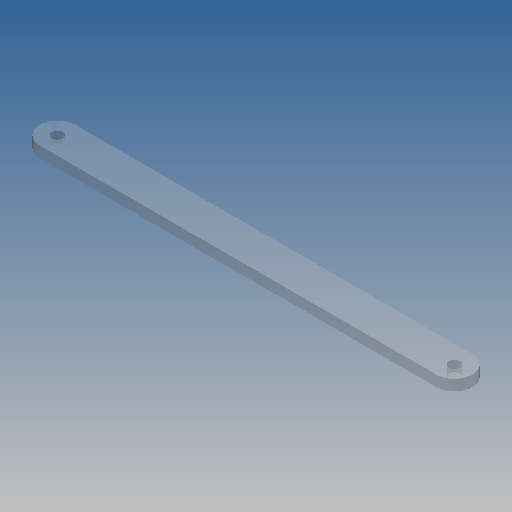
# Autodesk Inventor part: Handle
Saved by Autodesk Inventor 2017 (Build 210142000, 142)
## iProperties
Created: 2016-11-22
Part Number: Handle
Material: Polycarbonate, Clear
Document SubType Name: Modeling
Designer: James Yelland
Density: 1.2 g/cm^3
Appearance: Polycarbonate - Clear
Author: James Yelland
Autodesk Inventor part; units mm, degrees
ref_plane "YZ Plane" through (0, 0, 0) normal (1, 0, 0) x (0, 1, 0)
ref_plane "XZ Plane" through (0, 0, 0) normal (0, 1, 0) x (-1, 0, 0)
ref_plane "XY Plane" through (0, 0, 0) normal (0, 0, 1) x (1, 0, 0)
sketch "Sketch1" plane through (0, 0, 0) normal (0, 1, 0) x (-1, 0, 0)
  circle A0 centre (-55.4009, 75.9203) radius 1.6
  circle A1 centre (55.3868, 75.9203) radius 1.6
  arc A2 (55.3868, 70.9203) -> (55.3868, 80.9203) centre (55.3868, 75.9203) ccw
  line L0 (55.3868, 75.9203) -> (55.3868, 70.9203) construction
  line L1 (55.3868, 75.9203) -> (60.3868, 75.9203) construction
  line L2 (55.3868, 75.9203) -> (55.3868, 80.9203) construction
  arc A3 (-55.4009, 80.9203) -> (-55.4009, 70.9203) centre (-55.4009, 75.9203) ccw
  line L3 (-55.4009, 75.9203) -> (-50.4009, 75.9203) construction
  line L4 (-55.4009, 75.9203) -> (-55.4009, 80.9203) construction
  line L5 (-55.4009, 80.9203) -> (55.3868, 80.9203)
  line L6 (55.3868, 70.9203) -> (-55.4009, 70.9203)
  dimension "d13" = 5
  dimension "d14" = 90
  dimension "d15" = 180
  dimension "d16" = 5
  constraints: 14 end point, 4 centre point, 4 point on circle, 3 horizontal, 2 coincident, 1 perpendicular
  measures "d13" radius of A2
  measures "d14" angle of L0 L1
  measures "d15" angle of L0 L2
  measures "d16" radius of A3
extrude "Extrusion1" add sketch "Sketch1" along normal blind 3
body "Solid1"
